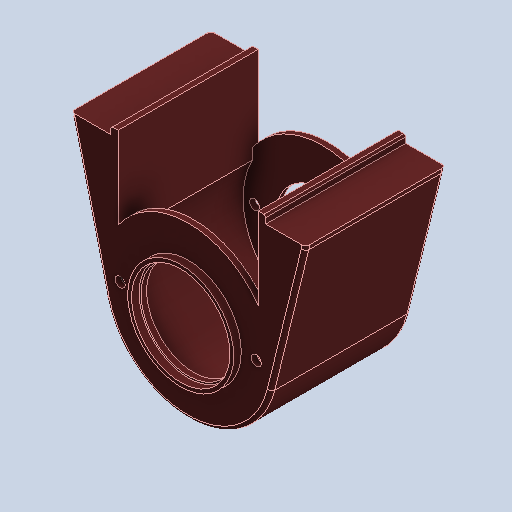
# Autodesk Inventor part: BodyStructure LumbarSupport
Saved by Autodesk Inventor 2023 (Build 270158000, 158)
## iProperties
Created: 2022-01-28
Part Number: BodyStructure LumbarSupport
Material: Generic
Document SubType Name: Modeling
Designer: Jochen
Density: 1 g/cm^3
Appearance: Default
Author: Jochen
Autodesk Inventor part; units mm, degrees
ref_plane "YZ Plane" through (0, 0, 0) normal (1, 0, 0) x (0, 1, 0)
ref_plane "XZ Plane" through (0, 0, 0) normal (0, 1, 0) x (-1, 0, 0)
ref_plane "XY Plane" through (0, 0, 0) normal (0, 0, 1) x (1, 0, 0)
sketch "Sketch1" plane through (0, 0, 0) normal (0, 0, 1) x (1, 0, 0)
  line L0 (0, -34.5) -> (0, 49.5) construction
  line L1 (-45.1691, 0) -> (45.1691, 0) construction
  circle A0 centre (0, 0) radius 13
  line L2 (18.5, 34) -> (-18.5, 34)
  line L3 (-18.5, 34) -> (-18.5, 12.8062)
  line L4 (18.5, 12.8062) -> (18.5, 34)
  circle A1 centre (0, 0) radius 22.5
  circle A2 centre (0, 0) radius 18 construction
  circle A3 centre (-18, 0) radius 1.325
  circle A4 centre (18, 0) radius 1.325
  line L5 (-27.638, 32.5) -> (27.638, 32.5)
  arc A5 (-32.2277, 37.5) -> (-32.0835, 36.3077) centre (-27.2277, 37.5) ccw construction
  line L6 (-32.2277, 37.5) -> (32.2277, 37.5) construction
  line L7 (-30.8558, 31.3077) -> (-21.8509, -5.3654)
  line L8 (30.8558, 31.3077) -> (23.1684, 0)
  arc A6 (-30.7984, 34) -> (-30.7766, 33.9779) centre (-27.2277, 37.5) ccw
  line L9 (23.1684, 0) -> (21.8509, -5.3654)
  arc A7 (32.0835, 36.3077) -> (32.2277, 37.5) centre (27.2277, 37.5) ccw construction
  line L10 (-27.638, 32.5) -> (-31.5216, 32.5)
  line L11 (27.638, 32.5) -> (31.5216, 32.5)
  arc A8 (-31, 32.5) -> (-30.8558, 31.3077) centre (-26, 32.5) ccw
  arc A9 (30.8558, 31.3077) -> (31, 32.5) centre (26, 32.5) ccw
  circle A10 centre (0, 0) radius 21
  line L12 (-21.8509, -5.3654) -> (-20.3942, -5.0077)
  line L13 (21.8509, -5.3654) -> (20.3942, -5.0077)
  line L14 (-18.5, 12.8062) -> (-17.2667, 11.9525)
  line L15 (18.5, 12.8062) -> (17.2667, 11.9525)
  line L16 (18.5, 12.8062) -> (18.5, 9.9373)
  line L17 (-18.5, 12.8062) -> (-18.5, 9.9373)
  point P0 (18.5, 32.5)
  point P1 (-18.5, 32.5)
  dimension "d2" = 26
  dimension "d17" = 45
  dimension "d18" = 37
  dimension "d19" = 34
  dimension "d20" = 36
  dimension "d21" = 2.65
  dimension "d25" = 32.5
  dimension "d27" = 5
  dimension "d34" = 62
  dimension "d35" = 5
  dimension "d36" = 1.5
  constraints: 32 end point, 23 point on circle, 13 tangent, 11 centre point, 7 point on line, 6 line through centre, 4 horizontal, 2 coincident, 2 equal radius, 2 parallel, 2 perpendicular, 1 vertical, 3 other
  measures "d2" diameter of A0
  measures "d17" diameter of A1
  measures "d18" distance of L2.start L2.end
  measures "d19" distance between parallel lines of L1 L2
  measures "d20" diameter of A2
  measures "d21" diameter of A3
  measures "d25" distance between parallel lines of L1 L5
  measures "d27" radius of A5
  measures "d34" distance of A8.start A9.end
  measures "d35" radius of A9
  measures "d36" radial gap between concentric circles of A1 A10
extrude "Extrusion1" add sketch "Sketch1" along normal blind 37 contours A0 | L15 A10 L14 A1 | L16 A10 L15 | A1 L13 A10 L16 | L17 A10 L12 A1 | L14 A10 L17 | A10 | L12 A10 L13 A1
extrude "Extrusion2" add sketch "Sketch1" along normal blind 20 separate body contours L15 A10 L14 A1 | L16 A10 L15 | A1 L13 A10 L16 | L17 A10 L12 A1 | L14 A10 L17 | A10 | L12 A10 L13 A1
combine bodies "Combine1" operation type add bodies to combine 2 1
ref_plane "Work Plane1" through (13.5, 34, 0) normal (0, 0, -1) x (-1, 0, 0)
sketch "Sketch2" plane through (13.5, 34, 0) normal (0, 0, -1) x (-1, 0, 0)
  circle A0 centre (13.5, -34) radius 14
  circle A1 centre (13.5, -34) radius 13 projected
  dimension "d10" = 28
  constraints: 1 centre point, 1 coincident
  measures "d10" diameter of A0
extrude "Extrusion3" add sketch "Sketch2" along normal blind 0.8 bodies 2
extrude "Extrusion4" add sketch "Sketch2" against normal blind 2 from surface at -37 bodies 2
shell "Shell2" thickness 1.5 removed faces 2 at (-1.5366, -1.6953, 37) at (-1.5366, -1.6953, 0) bodies 2
extrude "Extrusion5" add sketch "Sketch1" along normal up to surface (37 mm away) contours L5 L11 A9 L8 L9 A1 L4 | L3 A1 L7 A8 L10 L5 | L16 A10 L15 | A1 L13 A10 L16 | L17 A10 L12 A1 | L14 A10 L17 bodies 2
fillet "Fillet3" radius 1 9 edges at (-30.9638, 31.8995, 37) (-26.3533, 12.9712, 37) (30.9638, 31.8995, 37) (26.3533, 12.9712, 37) (0, -22.5, 0) (26.3533, 12.9712, 0) (30.9638, 31.8995, 0) (-30.9638, 31.8995, 0) (-26.3533, 12.9712, 0)
extrude "Extrusion6" cut sketch "Sketch1" along normal up to surface (34 mm away) from surface at 1.5 contours L15 A10 L14 A1 | L16 A10 L15 | L14 A10 L17 | A10 bodies 2
sketch "Sketch3" plane through (18.5, 32.5, 37) normal (0, 1, 0) x (1, 0, 0)
  arc A0 (12.5, 36) -> (11.5, 37) centre (11.5, 36) ccw projected
  line L0 (11.5, 37) -> (0, 37) projected
  line L1 (0, 37) -> (0, 0) projected
  line L2 (0, 0) -> (11.5, 0) projected
  arc A1 (11.5, 0) -> (12.5, 1) centre (11.5, 1) ccw projected
  line L3 (12.5, 36) -> (12.5, 1) projected
  arc A2 (-48.5, 37) -> (-49.5, 36) centre (-48.5, 36) ccw projected
  line L4 (-49.5, 36) -> (-49.5, 1) projected
  arc A3 (-49.5, 1) -> (-48.5, 0) centre (-48.5, 1) ccw projected
  line L5 (-48.5, 0) -> (-37, 0) projected
  line L6 (-37, 37) -> (-37, 0) projected
  line L7 (-37, 37) -> (-48.5, 37) projected
  line L8 (2.3798, 37) -> (11.3846, 37) projected
  line L9 (2, 37) -> (2, 0)
  line L10 (-39, 37) -> (-39, 0)
  point P0 (-18.5, 37)
  point P1 (2, 37)
  dimension "d39" = 2
  dimension "d40" = 2
  constraints: 4 end point, 4 point on line, 1 vertical
  measures "d39" distance between parallel lines of L9 L1
  measures "d40" distance between parallel lines of L10 L6
extrude "Extrusion7" add sketch "Sketch3" along normal blind 2 contours L2 L1 L0 L9 | L7 L6 L5 L10 bodies 2
chamfer "Chamfer2" distance 0.5 angle 45 2 edges at (20.5, 34.5, 18.5) (-20.5, 34.5, 18.5)
body "Solid2"
